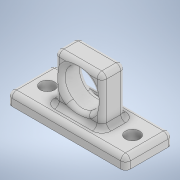
# Autodesk Inventor part: cable_holder
Saved by Autodesk Inventor 2021.4 (Build 254397000, 397)
## iProperties
Created: 2023-07-27
Part Number: cable_holder
Material: 一般
Document SubType Name: Modeling
Designer: ryusei
Density: 1 g/cm^3
Appearance: 既定
Author: ryusei
Autodesk Inventor part; units mm, degrees
ref_plane "YZ Plane" through (0, 0, 0) normal (1, 0, 0) x (0, 1, 0)
ref_plane "XZ Plane" through (0, 0, 0) normal (0, 1, 0) x (-1, 0, 0)
ref_plane "XY Plane" through (0, 0, 0) normal (0, 0, 1) x (1, 0, 0)
sketch "スケッチ1" plane through (0, 0, 0) normal (0, 1, 0) x (-1, 0, 0)
  line L0 (25, 10) -> (-25, 10)
  line L1 (-25, 10) -> (-25, -10)
  line L2 (-25, -10) -> (25, -10)
  line L3 (25, -10) -> (25, 10)
  line L4 (25, 10) -> (-25, -10) construction
  line L5 (-25, 10) -> (25, -10) construction
  point P0 (0, 0)
  dimension "d0" = 20
  dimension "d1" = 50
  constraints: 12 end point, 2 midpoint, 2 parallel, 1 horizontal, 1 perpendicular
  measures "d0" distance of L0.end L1.end
  measures "d1" distance of L1.end L2.end
extrude "押し出し1" add sketch "スケッチ1" along normal blind 5
sketch "スケッチ2" plane through (0, 5, 0) normal (0, 1, 0) x (1, 0, 0)
  line L0 (-10, -5) -> (10, -5)
  line L1 (10, -5) -> (10, 5)
  line L2 (10, 5) -> (-10, 5)
  line L3 (-10, 5) -> (-10, -5)
  line L4 (-10, -5) -> (10, 5) construction
  line L5 (10, -5) -> (-10, 5) construction
  point P0 (0, 0)
  dimension "d4" = 10
  dimension "d5" = 20
  constraints: 12 end point, 2 midpoint, 2 parallel, 1 horizontal, 1 perpendicular
  measures "d4" distance of L0.end L1.end
  measures "d5" distance of L1.end L2.end
extrude "押し出し2" add sketch "スケッチ2" along normal blind 20
sketch "スケッチ3" plane through (-10, 5, 5) normal (0, 0, 1) x (1, 0, 0)
  line L0 (0, 0) -> (0, 20) projected
  line L1 (0, 20) -> (20, 20) projected
  point P0 (10, -5)
  point P1 (10, 10)
  dimension "d8" = 10
  dimension "d9" = 10
  measures "d8" distance from line of L0 point (10, 10)
  measures "d9" distance from line of point (10, 10) L1
hole "穴1" at (0, 15, 5) direction (0, 0, -1) diameter 15 end through all
sketch "スケッチ4" plane through (0, 5, 0) normal (0, 1, 0) x (1, 0, 0)
  line L0 (-25, -10) -> (25, -10) projected
  line L1 (-25, 10) -> (-25, -10) projected
  line L2 (25, -10) -> (25, 10) projected
  point P0 (0, 0)
  point P1 (-18, 0)
  point P2 (18, 0)
  dimension "d17" = 10
  dimension "d18" = 7
  dimension "d19" = 7
  dimension "d20" = 10
  measures "d17" distance from line of L0 point (-18, 0)
  measures "d18" distance from line of L1 point (-18, 0)
  measures "d19" distance from line of L2 point (18, 0)
  measures "d20" distance from line of L0 point (18, 0)
hole "穴2" at (-18, 5, 0) at (18, 5, 0) direction (0, -1, 0) diameter 6 end through all
fillet "フィレット1" radius 2 22 edges at (0, 25, -5) (10, 25, 0) (10, 15, -5) (-10, 15, -5) (-10, 25, 0) (0, 25, 5) (10, 15, 5) (-10, 15, 5) (0, 5, 5) (-10, 5, 0) (0, 5, -5) (10, 5, 0) (0, 5, 10) (25, 5, 0) (0, 5, -10) (-25, 5, 0) (25, 2.5, -10) (-25, 2.5, -10) (25, 2.5, 10) (-25, 2.5, 10) (0, 22.5, -5) (0, 22.5, 5)
